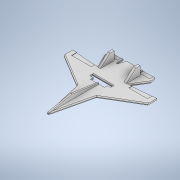
# Autodesk Inventor part: FIrst cad jet
Saved by Autodesk Inventor 2020 (Build 240168000, 168)
## iProperties
Created: 2019-05-11
Part Number: FIrst cad jet
Material: Generic
Document SubType Name: Modeling
Designer: kangh
Density: 1 g/cm^3
Appearance: Default
Author: kangh
Autodesk Inventor part; units mm, degrees
ref_plane "YZ Plane" through (0, 0, 0) normal (1, 0, 0) x (0, 1, 0)
ref_plane "XZ Plane" through (0, 0, 0) normal (0, 1, 0) x (-1, 0, 0)
ref_plane "XY Plane" through (0, 0, 0) normal (0, 0, 1) x (1, 0, 0)
sketch "Sketch1" plane through (0, 0, 0) normal (1, 0, 0) x (0, 1, 0)
  line L0 (5.08, 0) -> (5.08, 155.4155)
  line L1 (5.08, 155.4155) -> (0, 155.4155)
  line L2 (0, 155.4155) -> (0, -149.3845)
  line L3 (0, -149.3845) -> (5.08, -149.3845)
  line L4 (5.08, -149.3845) -> (5.08, 0)
  line L5 (5.08, 155.4155) -> (22.2119, 70.3851)
  line L6 (22.2119, 70.3851) -> (5.08, -52.858)
  line L7 (5.08, -77.8289) -> (36.3084, -113.2713)
  line L8 (36.3084, -113.2713) -> (36.3084, -128.1733)
  line L9 (36.3084, -128.1733) -> (5.08, -128.1733)
  point P0 (0, 0)
  dimension "d0" = 304.8
  dimension "d1" = 5.08
  constraints: 20 end point, 4 perpendicular, 4 point on line, 2 vertical, 1 collinear
  measures "d0" distance of L1.end L2.end
  measures "d1" distance of L1.end L0.end
extrude "Extrusion1" add sketch "Sketch1" along normal mid plane 304.8 contours L4 L3 L2 L1 L0
extrude "Extrusion2" add sketch "Sketch1" along normal mid plane 5.08 contours L0 L5 L6 L4
extrude "Extrusion3" add sketch "Sketch1" along normal mid plane 101.6 contours L7 L8 L9 L4
sketch "Sketch2" plane through (-50.8, 5.08, -77.8289) normal (0, 0.750304, 0.6610929) x (1, 0, 0)
  point P0 (50.8, -61.7537)
sketch "Sketch3" plane through (50.8, 36.3084, -128.1733) normal (0, 0, -1) x (-1, 0, 0)
  line L0 (101.6, 0) -> (0, 0) projected
  line L1 (101.6, -31.2284) -> (0, -31.2284) projected
  line L2 (8.8209, 0) -> (94.4146, 0)
  line L3 (94.4146, 0) -> (94.4146, -31.2284)
  line L4 (94.4146, -31.2284) -> (8.8209, -31.2284)
  line L5 (8.8209, -31.2284) -> (8.8209, 0)
  point P0 (50.8, -36.3084)
  constraints: 8 end point, 2 parallel, 2 point on line, 1 horizontal, 1 perpendicular
extrude "Extrusion4" cut sketch "Sketch3" against normal blind 101.6
sketch "Sketch4" plane through (-152.4, 5.08, -149.3845) normal (0, 1, 0) x (1, 0, 0)
  line L0 (0, -304.8) -> (149.86, -304.8) projected
  line L1 (149.86, -304.8) -> (116.9631, -164.6496)
  line L2 (116.9631, -164.6496) -> (0, -93.7758)
  line L3 (0, -93.7758) -> (0, -62.1552)
  line L4 (0, -304.8) -> (0, 0) projected
  line L5 (0, -62.1552) -> (94.6389, -69.5421)
  line L6 (94.6389, -69.5421) -> (72.8033, -22.902)
  line L7 (72.8033, -22.902) -> (74.5909, 0)
  line L8 (304.8, 0) -> (0, 0) projected
  point P0 (152.4, -149.3845)
  constraints: 12 end point, 3 point on line, 1 perpendicular
extrude "Extrusion5" cut sketch "Sketch4" against normal blind 101.6 contours L4 L2 L1 L0
extrude "Extrusion6" cut sketch "Sketch4" against normal mid plane 101.6 contours L4 L8 L7 L6 L5
sketch "Sketch5" plane through (152.4, 5.08, 155.4155) normal (0, 1, 0) x (1, 0, 0)
  line L0 (-187.8369, 140.1504) -> (-154.94, 0) projected
  line L1 (-154.94, 0) -> (-154.94, 181.9888) projected
  line L2 (-149.86, 181.9888) -> (-149.86, 0) projected
  line L3 (-116.9608, 140.1504) -> (-149.86, 0)
  line L4 (-304.8, 211.0242) -> (-304.8, 242.6448) projected
  line L5 (0, 304.8) -> (0, 0) projected
  line L6 (-116.9608, 140.1504) -> (0, 211.0242)
  line L7 (-94.6385, 235.2579) -> (0, 242.6448)
  line L8 (-231.9967, 281.898) -> (-210.1611, 235.2579) projected
  line L9 (-231.9967, 281.898) -> (-202.8544, 281.898)
  line L10 (-101.6, 283.5888) -> (-101.6, 233.2444) projected
  line L11 (-101.6, 283.5888) -> (-64.1738, 284.2138)
  line L12 (-64.1738, 284.2138) -> (-69.0059, 304.8)
  line L13 (-230.2091, 304.8) -> (0, 304.8) projected
  line L14 (-94.6385, 235.2579) -> (-64.1738, 284.2138)
  point P0 (-152.4, 155.4155)
  constraints: 14 end point, 3 point on line, 1 horizontal
extrude "Extrusion7" cut sketch "Sketch5" along normal mid plane 101.6
sketch "Sketch6" plane through (2.54, 5.08, 155.4155) normal (0, 1, 0) x (1, 0, 0)
  line L0 (-37.9769, 140.1504) -> (-5.08, 0) projected
  line L1 (-37.9769, 140.1504) -> (-5.08, 140.1504)
  line L2 (-5.08, 140.1504) -> (0, 140.1504)
  line L3 (0, 181.9888) -> (0, 0) projected
  line L4 (0, 140.1504) -> (32.8969, 140.1504)
  line L5 (0, 0) -> (149.86, 0) projected
  line L6 (32.8969, 140.1504) -> (0, 0)
  line L7 (0, 0) -> (32.8969, 140.1504)
  line L8 (32.8969, 140.1504) -> (149.86, 209.9338)
  line L9 (149.86, 0) -> (149.86, 242.6448) projected
  point P0 (-2.54, 155.4155)
  constraints: 12 end point, 3 point on line, 2 horizontal
extrude "Extrusion8" cut sketch "Sketch6" along normal mid plane 101.6 contours L6 L8 L9 L5
sketch "Sketch7" plane through (-2.54, 5.08, 155.4155) normal (0, 1, 0) x (1, 0, 0)
  line L0 (0, 181.9888) -> (5.08, 181.9888) projected
  line L1 (0, 181.9888) -> (-25.2643, 181.9888)
  line L2 (-25.2643, 181.9888) -> (-25.2643, 192.488)
  line L3 (-25.2643, 192.488) -> (-38.3487, 192.488)
  line L4 (-38.3487, 192.488) -> (-38.3487, 202.8464)
  line L5 (-38.3487, 202.8464) -> (36.8865, 202.8464)
  line L6 (36.8865, 202.8464) -> (36.8865, 192.488)
  line L7 (36.8865, 192.488) -> (25.4377, 192.488)
  line L8 (25.4377, 192.488) -> (25.4377, 181.9888)
  line L9 (25.4377, 181.9888) -> (5.08, 181.9888)
  point P0 (2.54, 155.4155)
  constraints: 18 end point, 7 perpendicular, 3 point on line, 1 horizontal
extrude "Extrusion9" cut sketch "Sketch7" along normal mid plane 101.6
sketch "Sketch8" plane through (-2.54, 5.08, 155.4155) normal (0, 1, 0) x (1, 0, 0)
  line L0 (-75.2691, 304.8) -> (85.9341, 304.8) projected
  line L1 (2.54, 304.8) -> (-16.5414, 304.8)
  line L2 (-16.5414, 304.8) -> (-24.7191, 278.6269)
  line L3 (-24.7191, 278.6269) -> (-29.786, 280.21)
  line L4 (-29.786, 280.21) -> (-29.786, 304.8)
  line L5 (2.54, 304.8) -> (22.7118, 304.8)
  line L6 (29.254, 280.21) -> (22.7118, 304.8)
  line L7 (29.254, 280.21) -> (37.1568, 280.21)
  line L8 (37.1568, 280.21) -> (37.1568, 304.8)
  point P0 (2.54, 155.4155)
  constraints: 16 end point, 5 point on line, 3 perpendicular, 1 parallel
extrude "Extrusion10" cut sketch "Sketch8" along normal mid plane 101.6 fills toward (37.1068, 292.505) open curves L8 L7 L6 L5 L1 L2 L3 L4
sketch "Sketch9" plane through (2.54, 0, 155.4155) normal (0.9735404, 0, 0.2285149) x (0.2285149, 0, -0.9735404)
  point P0 (150.7229, 0)
fillet "Fillet1" radius 3.175 7 edges at (-93.9184, 5.08, -20.1718) (93.9184, 5.08, -19.6266) (-18.9884, 5.08, 85.3403) (18.9884, 5.08, 85.3403) (72.9939, 5.08, -104.3203) (-68.6789, 5.08, -103.1624) (-3.2711, 5.08, -47.4309)
fillet "Fillet2" radius 3.175 1 edges at (0, 5.08, 155.4155)
sketch "Sketch10" plane through (-27.8043, 5.08, -26.5733) normal (0, 1, 0) x (1, 0, 0)
  line L0 (-124.5957, 60.656) -> (-29.9567, 53.2691) projected
  line L1 (-109.555, 59.482) -> (-109.555, 41.0337)
  line L2 (-109.555, 41.0337) -> (-38.167, 41.0337)
  line L3 (-38.167, 41.0337) -> (-38.167, 53.9099)
  point P0 (27.8043, -26.5733)
  constraints: 6 end point, 2 perpendicular, 2 point on line, 1 vertical
sketch "Sketch11" plane through (-27.8043, 5.08, -26.5733) normal (0, 1, 0) x (1, 0, 0)
  line L0 (25.2643, -181.9888) -> (30.3443, -181.9888) projected
  line L1 (27.8043, -181.9888) -> (27.8043, 123.4043)
  line L2 (30.3443, -96.9584) -> (30.3443, -179.4409) projected
  line L3 (85.5658, 53.2691) -> (180.2043, 60.656) projected
  line L4 (96.2866, 54.1059) -> (96.2866, 42.6218)
  line L5 (96.2866, 42.6218) -> (164.5032, 42.6218)
  line L6 (164.5032, 42.6218) -> (164.5032, 59.4305)
  point P0 (27.8043, -26.5733)
  constraints: 8 end point, 2 perpendicular, 2 point on line, 1 midpoint, 1 parallel, 1 vertical
extrude "Extrusion11" cut sketch "Sketch10" against normal blind 1.27
extrude "Extrusion12" cut sketch "Sketch11" against normal blind 1.27
sketch "Sketch12" plane through (-27.8043, 5.08, -26.5733) normal (0, 1, 0) x (1, 0, 0)
  line L0 (111.1984, 122.8112) -> (62.4211, 122.8112) projected
  line L1 (105.9589, 122.8112) -> (105.9589, 108.7392)
  line L2 (105.9589, 108.7392) -> (68.6314, 108.7392)
  line L3 (68.6314, 108.7392) -> (68.6314, 122.8112)
  line L4 (-4.5217, 122.8112) -> (-50.0048, 122.8112) projected
  line L5 (-11.4674, 122.8112) -> (-11.4674, 108.7392)
  line L6 (-11.4674, 108.7392) -> (-43.3514, 108.7392)
  line L7 (-43.3514, 108.7392) -> (-43.3514, 122.8112)
  point P0 (27.8043, -26.5733)
  constraints: 12 end point, 6 point on line, 3 perpendicular, 1 parallel, 1 vertical
extrude "Extrusion13" cut sketch "Sketch12" against normal blind 1.27 contours L5 L6 L7 L4
extrude "Extrusion14" cut sketch "Sketch12" against normal blind 1.27 contours L1 L2 L3 L0
body "Solid1"
